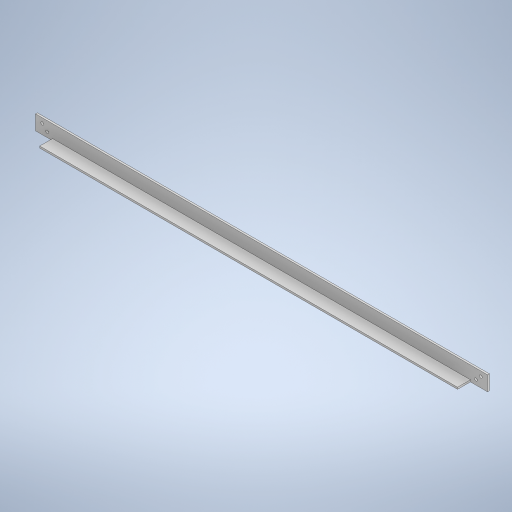
# Autodesk Inventor part: beamX
Saved by Autodesk Inventor 2023 (Build 270158000, 158)
## iProperties
Created: 2023-06-23
Part Number: beamX
Material: Generic
Document SubType Name: Modeling
Designer: incep
Density: 1 g/cm^3
Appearance: Default
Author: incep
Autodesk Inventor part; units mm, degrees
ref_plane "YZ Plane" through (0, 0, 0) normal (1, 0, 0) x (0, 1, 0)
ref_plane "XZ Plane" through (0, 0, 0) normal (0, 1, 0) x (-1, 0, 0)
ref_plane "XY Plane" through (0, 0, 0) normal (0, 0, 1) x (1, 0, 0)
sketch "Sketch1" plane through (0, 0, 0) normal (1, 0, 0) x (0, 1, 0)
  line L0 (25.4, 25.4) -> (0, 25.4) construction
  line L1 (0, 25.4) -> (0, 0)
  line L2 (0, 0) -> (25.4, 0)
  line L3 (25.4, 0) -> (25.4, 25.4) construction
  line L4 (25.4, 25.4) -> (3.175, 25.4) construction
  line L5 (3.175, 25.4) -> (3.175, 3.175)
  line L6 (3.175, 3.175) -> (25.4, 3.175)
  line L7 (25.4, 3.175) -> (25.4, 25.4) construction
  line L8 (25.4, 3.175) -> (25.4, 0)
  line L9 (3.175, 25.4) -> (0, 25.4)
  point P0 (0, 0)
  dimension "d1" = 25.4
  dimension "d2" = 3.175
  constraints: 20 end point, 5 perpendicular, 4 parallel, 2 horizontal, 1 coincident, 1 collinear
  measures "d1" distance of L0.start L0.end
  measures "d2" distance between parallel lines of L2 L6
extrude "Extrusion1" add sketch "Sketch1" along normal mid plane 781.15
sketch "Sketch2" plane through (-390.575, 3.175, 25.4) normal (0, 1, 0) x (1, 0, 0)
  line L0 (0, 0) -> (781.15, 0) projected
  line L1 (0, 0) -> (29.575, 0)
  line L2 (29.575, 0) -> (29.575, 22.225)
  line L3 (29.575, 22.225) -> (0, 22.225)
  line L4 (0, 22.225) -> (0, 0)
  line L5 (0, 22.225) -> (781.15, 22.225) projected
  point P0 (390.575, 25.4)
  point P1 (29.575, 0)
  dimension "d5" = 29.575
  constraints: 8 end point, 2 parallel, 1 horizontal, 1 perpendicular, 1 point on line
  measures "d5" distance between parallel lines of L2 L4
extrude "Extrusion2" cut sketch "Sketch2" against normal blind 3.175
sketch "Sketch3" plane through (-390.575, 25.4, 3.175) normal (0, 0, 1) x (1, 0, 0)
  line L0 (0, 0) -> (781.15, 0) construction
  line L1 (3.175, 0) -> (28.575, 0) construction
  line L2 (28.575, 0) -> (28.575, -25.4) construction
  line L3 (28.575, -25.4) -> (3.175, -25.4) construction
  line L4 (3.175, -25.4) -> (3.175, 0) construction
  line L5 (0, -25.4) -> (0, 0) construction
  line L6 (11.6417, -8.4667) -> (20.1083, -8.4667) construction
  line L7 (20.1083, -8.4667) -> (20.1083, -16.9333) construction
  line L8 (20.1083, -16.9333) -> (11.6417, -16.9333) construction
  line L9 (11.6417, -16.9333) -> (11.6417, -8.4667) construction
  circle A0 centre (11.6417, -8.4667) radius 2.4257
  circle A1 centre (20.1083, -16.9333) radius 2.4257
  point P0 (390.575, -25.4)
  point P1 (15.875, -8.4667)
  point P2 (15.875, 0)
  point P3 (20.1083, -12.7)
  point P4 (28.575, -12.7)
  dimension "d14" = 3.175
  dimension "d15" = 25.4
  dimension "d16" = 8.4667
  dimension "d17" = 4.8514
  constraints: 16 end point, 4 midpoint, 4 parallel, 4 perpendicular, 2 centre point, 2 coincident, 2 horizontal, 1 equal radius, 1 horizontal alignment, 1 point on line, 1 vertical alignment
  measures "d14" distance between parallel lines of L5 L4
  measures "d15" distance of L3.end L1.start
  measures "d16" distance of L6.start L6.end
  measures "d17" diameter of A0
extrude "Extrusion4" cut sketch "Sketch3" against normal blind 3.175
mirror "Mirror2" about plane through (0, 0, 0) normal (1, 0, 0) of "Extrusion4", "Extrusion2"
equation "\"d3\" = beamXW"
equation "\"d17\" = rivetHoleD"
equation "\"shelfMargin\" = 1"
equation "\"beamXW\" = 781.15"
equation "\"s_t\" = 3.175"
equation "\"rivetD\" = 4.7625"
equation "\"rivetHoleD\" = 4.8514"
body "Solid1"
